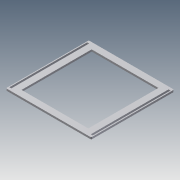
# Autodesk Inventor part: TopDiagonalPanel
Saved by Autodesk Inventor 2014 (Build 180170000, 170)
## iProperties
Created: 2014-08-11
Part Number: TopDiagonalPanel
Material: Generic
Document SubType Name: Modeling
Designer: Peele
Density: 1 g/cm^3
Appearance: White
Author: Peele
Autodesk Inventor part; units mm, degrees
ref_plane "YZ Plane" through (0, 0, 0) normal (1, 0, 0) x (0, 1, 0)
ref_plane "XZ Plane" through (0, 0, 0) normal (0, 1, 0) x (-1, 0, 0)
ref_plane "XY Plane" through (0, 0, 0) normal (0, 0, 1) x (1, 0, 0)
sketch "Sketch1" plane through (0, 0, 0) normal (0, 0, 1) x (1, 0, 0)
  line L0 (-134, -130.1931) -> (134, -130.1931)
  line L1 (134, -130.1931) -> (134, 130.1931)
  line L2 (134, 130.1931) -> (-134, 130.1931)
  line L3 (-134, 130.1931) -> (-134, -130.1931)
  line L4 (-134, -130.1931) -> (134, 130.1931) construction
  line L5 (134, -130.1931) -> (-134, 130.1931) construction
  point P0 (0, 0)
  dimension "d0" = 268
  dimension "d1" = 260.3863
  constraints: 12 end point, 2 midpoint, 2 parallel, 1 horizontal, 1 perpendicular
  measures "d0" distance of L0.start L0.end
  measures "d1" distance of L2.end L0.start
extrude "Extrusion1" add sketch "Sketch1" along normal blind 6
sketch "Sketch2" plane through (0, 0, 6) normal (0, 0, 1) x (1, 0, 0)
  line L0 (-134, -130.1931) -> (134, -130.1931) projected
  line L1 (134, 130.1931) -> (-134, 130.1931) projected
  line L2 (-134, 130.1931) -> (-134, -130.1931) projected
  line L3 (-131.125, 122.1931) -> (-124.875, 122.1931)
  line L4 (-124.875, 122.1931) -> (-124.875, -122.1931)
  line L5 (-124.875, -122.1931) -> (-131.125, -122.1931)
  line L6 (-131.125, -122.1931) -> (-131.125, 122.1931)
  line L7 (-131.125, 122.1931) -> (-124.875, -122.1931) construction
  line L8 (-124.875, 122.1931) -> (-131.125, -122.1931) construction
  point P0 (0, 0)
  point P1 (-128, 0)
  dimension "d5" = 2.875
  dimension "d6" = 6.25
  dimension "d7" = 8
  dimension "d101" = 8
  constraints: 12 end point, 2 midpoint, 2 parallel, 1 horizontal, 1 perpendicular
  measures "d5" distance between parallel lines of L2 L6
  measures "d6" distance of L3.start L3.end
  measures "d7" distance between parallel lines of L1 L3
  measures "d101" distance between parallel lines of L5 L0
extrude "Extrusion2" cut sketch "Sketch2" against normal through all
mirror "Mirror1" about plane through (0, 0, 0) normal (1, 0, 0) of "Extrusion2"
fillet "Fillet1" radius 3 4 edges at (134, 130.1931, 3) (134, -130.1931, 3) (-134, 130.1931, 3) (-134, -130.1931, 3)
sketch "Sketch3" plane through (0, 0, 6) normal (0, 0, 1) x (1, 0, 0)
  line L0 (131, 130.1931) -> (-131, 130.1931) projected
  line L1 (-124.875, 122.1931) -> (-124.875, -122.1931) projected
  line L2 (-104.875, -110.1931) -> (104.875, -110.1931)
  line L3 (104.875, -110.1931) -> (104.875, 110.1931)
  line L4 (104.875, 110.1931) -> (-104.875, 110.1931)
  line L5 (-104.875, 110.1931) -> (-104.875, -110.1931)
  line L6 (-104.875, -110.1931) -> (104.875, 110.1931) construction
  line L7 (104.875, -110.1931) -> (-104.875, 110.1931) construction
  point P0 (0, 0)
  dimension "d12" = 20
  dimension "d13" = 20
  constraints: 12 end point, 2 midpoint, 2 parallel, 1 horizontal, 1 perpendicular
  measures "d12" distance between parallel lines of L0 L4
  measures "d13" distance between parallel lines of L1 L5
extrude "Extrusion3" cut sketch "Sketch3" against normal through all
body "Solid1"
